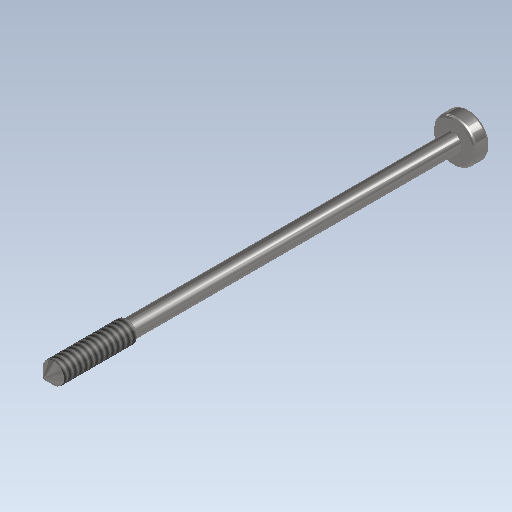
# Autodesk Inventor part: Длинный винт
Saved by Autodesk Inventor 2020 (Build 240168000, 168)
## iProperties
Created: 2018-08-28
Part Number: Длинный винт
Material: Сталь нержавеющая, 440C
Document SubType Name: Modeling
Designer: Shepelev
Density: 7.75 g/cm^3
Appearance: С умеренной полировкой
Author: Shepelev
Autodesk Inventor part; units mm, degrees
ref_plane "YZ Plane" through (0, 0, 0) normal (1, 0, 0) x (0, 1, 0)
ref_plane "XZ Plane" through (0, 0, 0) normal (0, 1, 0) x (-1, 0, 0)
ref_plane "XY Plane" through (0, 0, 0) normal (0, 0, 1) x (1, 0, 0)
sketch "Эскиз1" plane through (0, 0, 0) normal (1, 0, 0) x (0, 1, 0)
  line L0 (0, 20) -> (0.5, 20)
  line L1 (0.5, 20) -> (0.5, 16)
  line L2 (0.5, 16) -> (0.4, 16)
  line L3 (0.4, 16) -> (0.4, 0.75)
  line L4 (0.4, 0.75) -> (1, 0.75)
  line L5 (1, 0.75) -> (1, 0)
  line L6 (1, 0) -> (0, 0)
  line L7 (0, 0) -> (0, 20)
  line L8 (0, -4) -> (0, 24) projected
  dimension "d0" = 20
  dimension "d1" = 1
  dimension "d2" = 0.8
  dimension "d3" = 2
  dimension "d4" = 0.75
  dimension "d5" = 4
  constraints: 16 end point, 7 perpendicular, 1 horizontal
  measures "d0" distance of L6.end L0.start
  measures "d1" diameter of L1 L8
  measures "d2" diameter of L3 L8
  measures "d3" diameter of L5 L8
  measures "d4" distance of L4.end L5.end
  measures "d5" distance of L0.end L1.end
revolve "Вращение1" add sketch "Эскиз1" angle 360 about axis through (0, 0, -10) along (0, 0, 1)
thread "Резьба1" size "M1x0,25" class "6g" standard "ISO Metric profile" full length
chamfer "Фаска1" distance 0.5 angle 45 1 edges at (0, -0.5, 20)
chamfer "Фаска2" distance 0.1 angle 45 1 edges at (0, -0.5, 16)
fillet "Сопряжение1" radius 0.15 2 edges at (0, -1, 0.75) (0, -1, 0)
sketch "Эскиз2" plane through (0, 0, 0) normal (0, 0, -1) x (-1, 0, 0)
  line L0 (-0.2, 0.7) -> (0.2, 0.7)
  line L1 (0.2, 0.7) -> (0.2, -0.7)
  line L2 (0.2, -0.7) -> (-0.2, -0.7)
  line L3 (-0.2, -0.7) -> (-0.2, 0.7)
  line L4 (-0.2, 0.7) -> (0.2, -0.7) construction
  line L5 (0.2, 0.7) -> (-0.2, -0.7) construction
  line L6 (-0.7, 0.2) -> (0.7, 0.2)
  line L7 (0.7, 0.2) -> (0.7, -0.2)
  line L8 (0.7, -0.2) -> (-0.7, -0.2)
  line L9 (-0.7, -0.2) -> (-0.7, 0.2)
  line L10 (-0.7, 0.2) -> (0.7, -0.2) construction
  line L11 (0.7, 0.2) -> (-0.7, -0.2) construction
  line L12 (0, -1.4) -> (0, 1.4) projected
  line L13 (1.4, 0) -> (-1.4, 0) projected
  point P0 (0, 0)
  dimension "d16" = 0.4
  dimension "d17" = 0.4
  dimension "d18" = 1.4
  dimension "d19" = 1.4
  constraints: 24 end point, 4 midpoint, 4 parallel, 2 horizontal, 2 perpendicular, 4 other
  measures "d16" distance of L6.end L7.end
  measures "d17" distance of L1.end L2.end
  measures "d18" distance of L2.end L0.start
  measures "d19" distance of L7.end L8.end
extrude "Выдавливание1" cut sketch "Эскиз2" against normal blind 0.5
sketch "Эскиз3" plane through (0, 0, 0.5) normal (0, 0, -1) x (-1, 0, 0)
  line L0 (0.2, 0.7) -> (0.2, 0.2) projected
  line L1 (-0.2, -0.2) -> (0.2, -0.2)
  line L2 (0.2, -0.2) -> (0.2, 0.2)
  line L3 (0.2, 0.2) -> (-0.2, 0.2)
  line L4 (-0.2, 0.2) -> (-0.2, -0.2)
  line L5 (-0.2, -0.2) -> (0.2, 0.2) construction
  line L6 (0.2, -0.2) -> (-0.2, 0.2) construction
  point P0 (0, 0)
  constraints: 12 end point, 2 midpoint, 2 parallel, 1 horizontal, 1 perpendicular
extrude "Выдавливание2" cut sketch "Эскиз3" against normal blind 0.2
sketch "Эскиз4" plane through (0, 0, 0) normal (1, 0, 0) x (0, 1, 0)
  line L0 (0.2, 0.7) -> (-0.2, 0.7) projected
  line L1 (0.7, 0.5) -> (0.2, 0.5) projected
  line L2 (0.2, 0.7) -> (0.7, 0.5)
  line L3 (0.7, 0.5) -> (0.2, 0.5)
  line L4 (0.2, 0.5) -> (0.2, 0.7)
  line L5 (0.2, 0.5) -> (0.2, 0.7) projected
  point P0 (0, 0)
  constraints: 6 end point, 2 collinear, 1 point on line
extrude "Выдавливание3" cut sketch "Эскиз4" along normal mid plane 0.4
pattern_circular "Круговой массив1" count 4 over 360 about axis through (0, 0, 0.15) along (0, 0, -1) of "Выдавливание3"
chamfer "Фаска3" distance 0.1 angle 45 20 edges at (-0.2, 0.45, 0.6) (-0.45, 0.2, 0.6) (0.2, 0.45, 0.6) (0.45, 0.2, 0.6) (0.45, -0.2, 0.6) (0.2, -0.45, 0.6) (-0.45, -0.2, 0.6) (-0.2, -0.45, 0.6) (-0.2, 0.2, 0.35) (-0.2, -0.2, 0.35) (0.2, -0.2, 0.35) (0.2, 0.2, 0.35) (-0.2, 0.7, 0.25) (0.2, 0.7, 0.25) (0.7, 0.2, 0.25) (0.7, -0.2, 0.25) (0.2, -0.7, 0.25) (-0.2, -0.7, 0.25) (-0.7, -0.2, 0.25) (-0.7, 0.2, 0.25)
equation "\"d17\" = d16"
equation "\"d18\" = d19"
